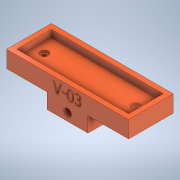
# Autodesk Inventor part: connectorToTubeBrackets03
Saved by Autodesk Inventor 2021.1 (Build 251245010, 245A)
## iProperties
Created: 2020-07-23
Part Number: connectorToTubeBrackets03
Material: PBT Plastic
Document SubType Name: Modeling
Designer: robst
Density: 1.31 g/cm^3
Appearance: Smooth - Light Orange
Mass: 251.144 g
Surface Area: 396.963 cm^2
Volume: 251.144 cm^3
Author: robst
Autodesk Inventor part; units mm, degrees
note: some values were not read from the file. Chosen so that the rebuilt part matches the saved one: direction of "Hole2"; direction of "Hole3"; direction of "Hole4".
ref_plane "YZ Plane" through (0, 0, 0) normal (1, 0, 0) x (0, 1, 0)
ref_plane "XZ Plane" through (0, 0, 0) normal (0, 1, 0) x (-1, 0, 0)
ref_plane "XY Plane" through (0, 0, 0) normal (0, 0, 1) x (1, 0, 0)
sketch "Sketch1" plane through (0, 0, 0) normal (0, 1, 0) x (-1, 0, 0)
  line L0 (69.85, 21.59) -> (-69.85, 21.59)
  line L1 (-69.85, 21.59) -> (-69.85, -21.59)
  line L2 (-69.85, -21.59) -> (69.85, -21.59)
  line L3 (69.85, -21.59) -> (69.85, 21.59)
  line L4 (69.85, 21.59) -> (-69.85, -21.59) construction
  line L5 (-69.85, 21.59) -> (69.85, -21.59) construction
  line L6 (76.2, 27.94) -> (-76.2, 27.94)
  line L7 (-76.2, 27.94) -> (-76.2, -27.94)
  line L8 (-76.2, -27.94) -> (76.2, -27.94)
  line L9 (76.2, -27.94) -> (76.2, 27.94)
  line L10 (76.2, 27.94) -> (-76.2, -27.94) construction
  line L11 (-76.2, 27.94) -> (76.2, -27.94) construction
  point P0 (0, 0)
  dimension "d0" = 43.18
  dimension "d1" = 139.7
  dimension "d2" = 6.35
  dimension "d3" = 6.35
  constraints: 24 end point, 4 midpoint, 4 parallel, 2 horizontal, 2 perpendicular
  measures "d0" distance of L0.end L1.end
  measures "d1" distance between parallel lines of L1 L3
  measures "d2" distance between parallel lines of L8 L2
  measures "d3" distance between parallel lines of L9 L3
extrude "Extrusion1" add sketch "Sketch1" against normal blind 12.065 contours L3 L2 L1 L0 | L9 L8 L7 L6
extrude "Extrusion2" add sketch "Sketch1" along normal blind 8.89
sketch "Sketch2" plane through (0, 0, 0) normal (0, 1, 0) x (1, 0, 0)
  line L0 (-69.85, 21.59) -> (-69.85, -21.59) construction
  line L1 (-69.85, 0) -> (69.85, 0) construction
  line L2 (69.85, -21.59) -> (69.85, 21.59) construction
  point P0 (0, 0)
  point P1 (-57.15, 0)
  point P2 (57.15, 0)
  dimension "d8" = 12.7
  dimension "d9" = 12.7
  constraints: 2 end point, 2 midpoint, 2 point on line
  measures "d8" distance from line of point (-57.15, 0) L0
  measures "d9" distance from line of point (57.15, 0) L2
hole "Hole1" at (-57.15, 0, 0) at (57.15, 0, 0) direction (0, -1, 0) diameter 5.1054 end through all counterbore diameter 10.16 counterbore depth 2.54 clearance for "Hex Machine Screw" size "#10" standard "Ansi Unified Screw Threads"
sketch "Sketch5" plane through (0, -12.065, 0) normal (0, -1, 0) x (1, 0, 0)
  line L0 (-25.4, -27.94) -> (25.4, -27.94)
  line L1 (25.4, -27.94) -> (25.4, 27.94)
  line L2 (25.4, 27.94) -> (-25.4, 27.94)
  line L3 (-25.4, 27.94) -> (-25.4, -27.94)
  line L4 (-25.4, -27.94) -> (25.4, 27.94) construction
  line L5 (25.4, -27.94) -> (-25.4, 27.94) construction
  point P0 (0, 0)
  dimension "d27" = 50.8
  dimension "d28" = 55.88
  constraints: 12 end point, 2 midpoint, 2 parallel, 1 horizontal, 1 perpendicular
  measures "d27" distance between parallel lines of L1 L3
  measures "d28" distance between parallel lines of L0 L2
extrude "Extrusion6" add sketch "Sketch5" along normal blind 19.05
sketch "Sketch6" plane through (-76.2, -12.065, 27.94) normal (0, 0, 1) x (1, 0, 0)
  line L0 (50.8, 0) -> (50.8, -19.05) projected
  line L1 (101.6, 0) -> (101.6, -19.05) projected
  line L2 (101.6, -19.05) -> (50.8, -19.05) projected
  line L3 (0, 20.955) -> (152.4, 20.955) projected
  line L4 (0, 0) -> (0, 20.955) projected
  line L5 (50.8, 0) -> (0, 0) projected
  line L6 (50.8, 0) -> (50.8, -19.05) projected
  line L7 (101.6, -19.05) -> (50.8, -19.05) projected
  line L8 (101.6, 0) -> (101.6, -19.05) projected
  line L9 (152.4, 0) -> (101.6, 0) projected
  line L10 (152.4, 20.955) -> (152.4, 0) projected
  line L11 (0, 0) -> (50.8, 0) construction
  line L12 (101.6, 0) -> (152.4, 0) construction
  circle A0 centre (76.2, -9.525) radius 4.7625
  point P0 (76.2, 12.065)
  dimension "d31" = 9.525
  dimension "d34" = 9.525
  dimension "d35" = 25.4
  constraints: 1 centre point
  measures "d31" diameter of A0
  measures "d34" distance from line of A0.centre L2
  measures "d35" distance from line of A0.centre L0
extrude "Extrusion7" cut sketch "Sketch6" against normal through all contours A0
sketch "Sketch7" plane through (0, -31.115, 0) normal (0, -1, 0) x (1, 0, 0)
  line L0 (76.2, -27.94) -> (-76.2, -27.94) construction
  line L1 (0, -27.94) -> (0, 27.94) construction
  line L2 (-76.2, 27.94) -> (76.2, 27.94) construction
  point P0 (0, 0)
  point P1 (0, -9.3133)
  point P2 (0, 9.3133)
  dimension "d36" = 18.6267
  dimension "d39" = 18.6267
  constraints: 2 end point, 2 midpoint, 1 point on line, 1 vertical, 1 other
  measures "d36" distance from line of point (0, -9.313) L0
  measures "d39" distance of point (0, -9.313) point (0, 9.313)
hole "Hole2" at (0, -31.115, -9.3133) at (0, -31.115, 9.3133) direction (0, 1, 0) diameter 5.1054 end up to surface counterbore diameter 6.5278 counterbore depth 6.35 clearance for "Hex Machine Screw" size "#10" standard "Ansi Unified Screw Threads"
sketch "Sketch9" plane through (-25.4, -12.065, -27.94) normal (-1, 0, 0) x (0, 0, 1)
  line L0 (0, 0) -> (0, -19.05) construction
  line L1 (0, -9.525) -> (55.88, -9.525) construction
  line L2 (55.88, 0) -> (55.88, -19.05) construction
  line L3 (55.88, -19.05) -> (0, -19.05) projected
  point P0 (27.94, 12.065)
  point P1 (18.6267, -9.525)
  point P2 (37.2533, -9.525)
  dimension "d60" = 9.525
  dimension "d61" = 18.6267
  dimension "d64" = 18.6267
  constraints: 2 end point, 2 horizontal, 2 midpoint, 1 point on line, 1 other
  measures "d60" distance between parallel lines of L1 L3
  measures "d61" distance from line of point (18.627, -9.525) L0
  measures "d64" distance of point (18.627, -9.525) point (37.253, -9.525)
hole "Hole3" at (-25.4, -21.59, -9.3133) at (-25.4, -21.59, 9.3133) direction (1, 0, 0) diameter 5.1054 end up to surface counterbore diameter 6.5278 counterbore depth 9.525 clearance for "Hex Machine Screw" size "#10" standard "Ansi Unified Screw Threads"
sketch "Sketch10" plane through (25.4, -12.065, 27.94) normal (1, 0, 0) x (0, 0, -1)
  line L0 (0, 0) -> (0, -19.05) construction
  line L1 (0, -9.525) -> (55.88, -9.525) construction
  line L2 (55.88, 0) -> (55.88, -19.05) construction
  line L3 (55.88, -19.05) -> (0, -19.05) projected
  circle A0 centre (18.6267, -9.525) radius 3.2639 projected
  circle A1 centre (37.2533, -9.525) radius 3.2639 projected
  point P0 (27.94, 12.065)
  dimension "d76" = 9.525
  constraints: 2 coincident, 2 end point, 2 midpoint, 1 horizontal
  measures "d76" distance between parallel lines of L1 L3
hole "Hole4" at (25.4, -21.59, 9.3133) at (25.4, -21.59, -9.3133) direction (-1, 0, 0) diameter 5.1054 end up to surface counterbore diameter 6.5278 counterbore depth 9.525 clearance for "Hex Machine Screw" size "#10" standard "Ansi Unified Screw Threads"
sketch "Sketch11" plane through (-76.2, 8.89, 27.94) normal (0, 0, 1) x (1, 0, 0)
  line L0 (0, -20.955) -> (0, 0) construction
  line L1 (0, -10.4775) -> (152.4, -10.4775) construction
  line L2 (152.4, 0) -> (152.4, -20.955) construction
  line L3 (68.7848, -4.1275) -> (64.4108, -16.8275)
  line L4 (64.4108, -16.8275) -> (62.5892, -16.8275)
  line L5 (62.5892, -16.8275) -> (58.2152, -4.1275)
  line L6 (58.2152, -4.1275) -> (60.0265, -4.1275)
  line L7 (60.0265, -4.1275) -> (63.5463, -14.6765)
  line L8 (63.5463, -14.6765) -> (67.0661, -4.1275)
  line L9 (67.0661, -4.1275) -> (68.7848, -4.1275)
  line L10 (74.435, -12.0418) -> (69.6287, -12.0418)
  line L11 (69.6287, -12.0418) -> (69.6287, -10.4981)
  line L12 (69.6287, -10.4981) -> (74.435, -10.4981)
  line L13 (74.435, -10.4981) -> (74.435, -12.0418)
  spline S0 degree 2 poles (84.0269, -10.4775) (84.0269, -13.8944) (82.0406, -17.0951) (79.9719, -17.0951) knots 0 0 0 1 2 2 2
  spline S1 degree 2 poles (79.9719, -17.0951) (77.8724, -17.0951) (75.9067, -13.8326) (75.9067, -10.4878) knots 0 0 0 1 2 2 2
  spline S2 degree 2 poles (75.9067, -10.4878) (75.9067, -7.0504) (77.893, -3.8702) (79.9719, -3.8702) knots 0 0 0 1 2 2 2
  spline S3 degree 2 poles (79.9719, -3.8702) (82.0611, -3.8702) (84.0269, -7.1636) (84.0269, -10.4775) knots 0 0 0 1 2 2 2
  spline S4 degree 2 poles (81.845, -14.3472) (82.092, -13.7194) (82.2979, -11.7846) (82.2979, -10.4775) knots 0 0 0 1 2 2 2
  spline S5 degree 2 poles (82.2979, -10.4775) (82.2979, -9.1704) (82.092, -7.2459) (81.8347, -6.5975) knots 0 0 0 1 2 2 2
  spline S6 degree 2 poles (81.8347, -6.5975) (81.5774, -5.9491) (80.6821, -5.2802) (79.9719, -5.2802) knots 0 0 0 1 2 2 2
  spline S7 degree 2 poles (79.9719, -5.2802) (79.2618, -5.2802) (78.3458, -5.9491) (78.0782, -6.6181) knots 0 0 0 1 2 2 2
  spline S8 degree 2 poles (78.0782, -6.6181) (77.8209, -7.2665) (77.6357, -9.2425) (77.6357, -10.4878) knots 0 0 0 1 2 2 2
  spline S9 degree 2 poles (77.6357, -10.4878) (77.6357, -11.8257) (77.8004, -13.6165) (78.068, -14.3163) knots 0 0 0 1 2 2 2
  spline S10 degree 2 poles (78.068, -14.3163) (78.315, -14.975) (79.2309, -15.6851) (79.9719, -15.6851) knots 0 0 0 1 2 2 2
  spline S11 degree 2 poles (79.9719, -15.6851) (80.6718, -15.6851) (81.5877, -15.0162) (81.845, -14.3472) knots 0 0 0 1 2 2 2
  spline S12 degree 2 poles (89.0801, -5.3316) (88.617, -5.3316) (87.701, -5.5581) (87.2585, -5.733) knots 0 0 0 1 2 2 2
  spline S13 degree 2 poles (87.2585, -5.733) (86.8468, -5.908) (86.2396, -6.2785) (86.0029, -6.4431) knots 0 0 0 1 2 2 2
  line L14 (86.0029, -6.4431) -> (85.9, -6.4431)
  line L15 (85.9, -6.4431) -> (85.9, -4.6421)
  spline S14 degree 2 poles (85.9, -4.6421) (86.4557, -4.3436) (88.3597, -3.8599) (89.2139, -3.8599) knots 0 0 0 1 2 2 2
  spline S15 degree 2 poles (89.2139, -3.8599) (90.0784, -3.8599) (91.3649, -4.2098) (91.8897, -4.5803) knots 0 0 0 1 2 2 2
  spline S16 degree 2 poles (91.8897, -4.5803) (92.4455, -4.9817) (93.0218, -6.1447) (93.0218, -6.9269) knots 0 0 0 1 2 2 2
  spline S17 degree 2 poles (93.0218, -6.9269) (93.0218, -7.9766) (91.6427, -9.5615) (90.6753, -9.7674) knots 0 0 0 1 2 2 2
  line L16 (90.6753, -9.7674) -> (90.6753, -9.8909)
  spline S18 degree 2 poles (90.6753, -9.8909) (91.0767, -9.9732) (91.9927, -10.3437) (92.3838, -10.7142) knots 0 0 0 1 2 2 2
  spline S19 degree 2 poles (92.3838, -10.7142) (92.7748, -11.0744) (93.2688, -12.2271) (93.2688, -13.0607) knots 0 0 0 1 2 2 2
  spline S20 degree 2 poles (93.2688, -13.0607) (93.2688, -13.9149) (92.6822, -15.3661) (92.147, -15.9218) knots 0 0 0 1 2 2 2
  spline S21 degree 2 poles (92.147, -15.9218) (91.5913, -16.4982) (90.0167, -17.0951) (89.0184, -17.0951) knots 0 0 0 1 2 2 2
  spline S22 degree 2 poles (89.0184, -17.0951) (88.0612, -17.0951) (86.1881, -16.632) (85.55, -16.3129) knots 0 0 0 1 2 2 2
  line L17 (85.55, -16.3129) -> (85.55, -14.5119)
  line L18 (85.55, -14.5119) -> (85.6735, -14.5119)
  spline S23 degree 2 poles (85.6735, -14.5119) (86.2087, -14.9029) (88.0201, -15.6234) (88.9154, -15.6234) knots 0 0 0 1 2 2 2
  spline S24 degree 2 poles (88.9154, -15.6234) (89.4403, -15.6234) (90.4901, -15.294) (90.84, -14.9132) knots 0 0 0 1 2 2 2
  spline S25 degree 2 poles (90.84, -14.9132) (91.1796, -14.5324) (91.5398, -13.6268) (91.5398, -12.9372) knots 0 0 0 1 2 2 2
  spline S26 degree 2 poles (91.5398, -12.9372) (91.5398, -12.2477) (91.1385, -11.3523) (90.7782, -11.095) knots 0 0 0 1 2 2 2
  spline S27 degree 2 poles (90.7782, -11.095) (90.418, -10.8377) (89.4403, -10.6422) (88.864, -10.6422) knots 0 0 0 1 2 2 2
  line L19 (88.864, -10.6422) -> (88.1436, -10.6422)
  line L20 (88.1436, -10.6422) -> (88.1436, -9.2322)
  line L21 (88.1436, -9.2322) -> (88.7096, -9.2322)
  spline S28 degree 2 poles (88.7096, -9.2322) (89.852, -9.2322) (91.2928, -8.1413) (91.2928, -7.1018) knots 0 0 0 1 2 2 2
  spline S29 degree 2 poles (91.2928, -7.1018) (91.2928, -6.6181) (90.9223, -5.9286) (90.6239, -5.7227) knots 0 0 0 1 2 2 2
  spline S30 degree 2 poles (90.6239, -5.7227) (90.3048, -5.5066) (89.5226, -5.3316) (89.0801, -5.3316) knots 0 0 0 1 2 2 2
  point P0 (76.2, -8.89)
  constraints: 2 end point, 2 midpoint, 1 horizontal
extrude "Extrusion8" cut sketch "Sketch11" against normal blind 2.54
equation "\"d0\" = innerWidth"
equation "\"d1\" = innerLength"
equation "\"d2\" = wallThickness"
equation "\"d3\" = wallThickness"
equation "\"d4\" = bottomThickness"
equation "\"d6\" = innerDepth"
equation "\"d8\" = holeCenterFromInnerWall"
equation "\"d9\" = holeCenterFromInnerWall"
equation "\"d27\" = lowerPostLength"
equation "\"d28\" = lowerPostWidth"
equation "\"d29\" = lowerPostHeight"
equation "\"d31\" = postDiameter"
equation "\"d34\" = lowerPostCenterY"
equation "\"d35\" = 0.5 * lowerPostLength"
equation "\"d36\" = setScrewCenters"
equation "\"d39\" = setScrewCenters"
equation "\"d60\" = lowerPostCenterY"
equation "\"d61\" = setScrewCenters"
equation "\"d64\" = setScrewCenters"
equation "\"d76\" = lowerPostCenterY"
equation "\"innerWidth\" = 43.18"
equation "\"innerLength\" = 139.7"
equation "\"innerDepth\" = 8.89"
equation "\"wallThickness\" = 6.35"
equation "\"postDiameter\" = 9.525"
equation "\"holeCenterFromInnerWall\" = 12.7"
equation "\"bottomThickness\" = 12.065"
equation "\"d17\" = postDiameter"
equation "\"exteriorWidth\" = innerWidth + 2 * wallThickness"
equation "\"exteriorLength\" = innerLength + 2 * wallThickness"
equation "\"exteriorHeight\" = innerDepth + bottomThickness"
equation "\"d24\" = postDiameter"
equation "\"lowerPostWidth\" = exteriorWidth"
equation "\"lowerPostLength\" = 50.8"
equation "\"lowerPostCenterX\" = 0.5 * exteriorLength"
equation "\"lowerPostHeight\" = 19.05"
equation "\"lowerPostCenterY\" = postDiameter"
equation "\"setScrewCenters\" = 0.333333 * exteriorWidth"
body "Solid1"
